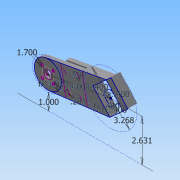
# Autodesk Inventor part: MountSketch
Saved by Autodesk Inventor 2014 SP1 (Build 180222100, 222)
## iProperties
Created: 2014-05-16
Part Number: MountSketch
Material: Generic
Document SubType Name: Modeling
Designer: dliu
Density: 1 g/cm^3
Appearance: Default
Author: dliu
Autodesk Inventor part; units mm, degrees
ref_plane "Back Plane" through (0, 0, -12.7) normal (0, 0, -1) x (-1, 0, 0)
ref_plane "Midplane" through (0, 0, -6.35) normal (0, 0, 1) x (1, 0, 0)
ref_plane "YZ Plane" through (0, 0, 0) normal (1, 0, 0) x (0, 1, 0)
sketch "the Axle" plane through (0, 0, 0) normal (0, 0, 1) x (1, 0, 0)
  line L0 (-30.4731, 63.7704) -> (-43.9693, 51.6183)
  line L1 (-43.9693, 51.6183) -> (-54.1341, 62.9075)
  line L2 (-40.6378, 75.0595) -> (-30.4731, 63.7704)
  line L3 (-30.4731, 63.7704) -> (-12.3121, 63.7704) construction
  arc A0 (-40.6378, 75.0595) -> (-54.1341, 62.9075) centre (-42.9621, 64.0703) ccw
  line L4 (-54.1341, 62.9075) -> (-40.6378, 75.0595) construction
  point P0 (-12.6671, 65.6222)
  dimension "d84" = 18.161
  dimension "d85" = 138
  dimension "d231" = 19.812
  measures "d84" distance of L2.end L1.start
  measures "d85" angle of L0 L3
sketch "Motor Mount Pattern" plane through (0, 0, 0) normal (0, 0, 1) x (1, 0, 0)
  line L0 (-116.3697, 51.2894) -> (-116.3697, 68.9671) construction
  line L1 (-116.3697, 68.9671) -> (-134.0474, 68.9671) construction
  line L2 (-134.0474, 68.9671) -> (-134.0474, 51.2894) construction
  line L3 (-134.0474, 51.2894) -> (-116.3697, 68.9671) construction
  line L4 (-116.3697, 51.2894) -> (-134.0474, 68.9671) construction
  line L5 (-134.0474, 51.2894) -> (-134.0474, 68.9671) construction
  line L6 (-134.0474, 51.2894) -> (-116.3697, 68.9671) construction
  line L7 (-134.0474, 51.2894) -> (-125.2086, 60.1282) construction
  line L8 (-116.3697, 51.2894) -> (-134.0474, 51.2894) construction
  circle A0 centre (-125.2086, 60.1282) radius 6.2
  circle A1 centre (-116.3697, 68.9671) radius 2.25
  circle A2 centre (-134.0474, 68.9671) radius 2.25
  circle A3 centre (-116.3697, 51.2894) radius 2.25
  circle A4 centre (-134.0474, 51.2894) radius 2.25
  circle A5 centre (-116.3697, 68.9671) radius 4.5 construction
  circle A6 centre (-134.0474, 68.9671) radius 4.5 construction
  circle A7 centre (-134.0474, 51.2894) radius 4.5 construction
  circle A8 centre (-116.3697, 51.2894) radius 4.5 construction
  point P0 (-121.7102, 57.8126)
  dimension "d189" = 25
  dimension "d192" = 12.4
  dimension "d193" = 4.5
  dimension "d195" = 9
  measures "d189" distance of L0.start L1.end
  measures "d192" diameter of A0
  measures "d193" diameter of A1
  measures "d195" diameter of A5
sketch "Motor Body Extent" plane through (0, 0, 0) normal (0, 0, 1) x (1, 0, 0)
  circle A0 centre (-176.4641, 62.233) radius 24.5 construction
  dimension "MotorDia" = 49
  measures "MotorDia" diameter of A0
sketch "Block7" plane through (0, 0, 0) normal (0, 0, 1) x (1, 0, 0)
  line L0 (-114.6206, 39.8537) -> (-104.0422, 54.0169) construction
  line L1 (-104.0422, 54.0169) -> (-118.2054, 64.5953) construction
  line L2 (-118.2054, 64.5953) -> (-128.7838, 50.432) construction
  line L3 (-128.7838, 50.432) -> (-104.0422, 54.0169) construction
  line L4 (-114.6206, 39.8537) -> (-118.2054, 64.5953) construction
  line L5 (-128.7838, 50.432) -> (-118.2054, 64.5953) construction
  line L6 (-128.7838, 50.432) -> (-104.0422, 54.0169) construction
  line L7 (-128.7838, 50.432) -> (-116.413, 52.2245) construction
  line L8 (-114.6206, 39.8537) -> (-128.7838, 50.432) construction
  circle A0 centre (-116.413, 52.2245) radius 6.2
  circle A1 centre (-104.0422, 54.0169) radius 2.25
  circle A2 centre (-118.2054, 64.5953) radius 2.25
  circle A3 centre (-114.6206, 39.8537) radius 2.25
  circle A4 centre (-128.7838, 50.432) radius 2.25
  circle A5 centre (-104.0422, 54.0169) radius 4.5 construction
  circle A6 centre (-118.2054, 64.5953) radius 4.5 construction
  circle A7 centre (-128.7838, 50.432) radius 4.5 construction
  circle A8 centre (-114.6206, 39.8537) radius 4.5 construction
  line L9 (-107.5171, 56.2696) -> (-121.6653, 66.8681) construction
  line L10 (-121.6653, 66.8681) -> (-132.2638, 52.7199) construction
  line L11 (-132.2638, 52.7199) -> (-118.1156, 42.1214) construction
  line L12 (-118.1156, 42.1214) -> (-121.6653, 66.8681) construction
  line L13 (-107.5171, 56.2696) -> (-132.2638, 52.7199) construction
  line L14 (-118.1156, 42.1214) -> (-132.2638, 52.7199) construction
  line L15 (-118.1156, 42.1214) -> (-121.6653, 66.8681) construction
  line L16 (-118.1156, 42.1214) -> (-119.8904, 54.4948) construction
  line L17 (-107.5171, 56.2696) -> (-118.1156, 42.1214) construction
  circle A9 centre (-119.8904, 54.4948) radius 6.2
  circle A10 centre (-121.6653, 66.8681) radius 2.25
  circle A11 centre (-132.2638, 52.7199) radius 2.25
  circle A12 centre (-107.5171, 56.2696) radius 2.25
  circle A13 centre (-118.1156, 42.1214) radius 2.25
  circle A14 centre (-121.6653, 66.8681) radius 4.5 construction
  circle A15 centre (-132.2638, 52.7199) radius 4.5 construction
  circle A16 centre (-118.1156, 42.1214) radius 4.5 construction
  circle A17 centre (-107.5171, 56.2696) radius 4.5 construction
  line L18 (-105.811, 55.3186) -> (-120.0113, 65.8472) construction
  line L19 (-120.0113, 65.8472) -> (-130.5399, 51.6469) construction
  line L20 (-130.5399, 51.6469) -> (-116.3396, 41.1183) construction
  line L21 (-116.3396, 41.1183) -> (-120.0113, 65.8472) construction
  line L22 (-105.811, 55.3186) -> (-130.5399, 51.6469) construction
  line L23 (-116.3396, 41.1183) -> (-130.5399, 51.6469) construction
  line L24 (-116.3396, 41.1183) -> (-120.0113, 65.8472) construction
  line L25 (-116.3396, 41.1183) -> (-118.1755, 53.4828) construction
  line L26 (-105.811, 55.3186) -> (-116.3396, 41.1183) construction
  circle A18 centre (-118.1755, 53.4828) radius 6.2
  circle A19 centre (-120.0113, 65.8472) radius 2.25
  circle A20 centre (-130.5399, 51.6469) radius 2.25
  circle A21 centre (-105.811, 55.3186) radius 2.25
  circle A22 centre (-116.3396, 41.1183) radius 2.25
  circle A23 centre (-120.0113, 65.8472) radius 4.5 construction
  circle A24 centre (-130.5399, 51.6469) radius 4.5 construction
  circle A25 centre (-116.3396, 41.1183) radius 4.5 construction
  circle A26 centre (-105.811, 55.3186) radius 4.5 construction
  point P0 (-115.0557, 53.032)
sketch "MotorMountPattern" plane through (0, 0, 0) normal (0, 0, 1) x (1, 0, 0)
  line L0 (-95.4079, 16.8905) -> (-77.7418, 16.8905) construction
  line L1 (-77.7418, 16.8905) -> (-77.7418, 34.5797) construction
  line L2 (-77.7418, 34.5797) -> (-95.4079, 34.5797) construction
  line L3 (-95.4079, 34.5797) -> (-95.4079, 16.8905) construction
  line L4 (-95.4079, 16.8905) -> (-77.7418, 34.5797) construction
  line L5 (-77.7418, 16.8905) -> (-95.4079, 34.5797) construction
  circle A0 centre (-95.4079, 34.5797) radius 2.2
  circle A1 centre (-77.7418, 34.5797) radius 2.2
  circle A2 centre (-77.7418, 16.8905) radius 2.2
  circle A3 centre (-95.4079, 16.8905) radius 2.2
  circle A4 centre (-86.5749, 25.7351) radius 6.35
  point P0 (-86.5749, 25.7351)
  dimension "d197" = 25
  dimension "M4Clearance" = 4.4
  dimension "MotorShaftClearance" = 12.7
  measures "d197" distance of L0.start L1.end
  measures "M4Clearance" diameter of A0
  measures "MotorShaftClearance" diameter of A4
sketch "Base Sketch" plane through (0, 0, 0) normal (0, 0, 1) x (1, 0, 0)
  line L0 (26.8378, -1.0519) -> (-1.7592, -26.8007)
  line L1 (-1.7592, -26.8007) -> (-28.6127, 3.0232)
  line L2 (-28.6127, 3.0232) -> (-0.0158, 28.772)
  line L3 (-0.0158, 28.772) -> (26.8378, -1.0519)
  line L4 (-7.5661, 21.9736) -> (19.2874, -7.8503)
  circle A0 centre (0, 0) radius 41.5 construction
  line L5 (-7.5661, 21.9736) -> (-79.8206, 8.7754)
  line L6 (-97.8004, -38.3626) -> (-71.7823, -35.2304)
  circle A1 centre (-100.3809, -16.9274) radius 21.59
  line L7 (-148.6125, -66.8274) -> (67.2297, -66.8274) construction
  circle A2 centre (-100.3809, -16.9274) radius 24.5 construction
  line L8 (-71.1528, -2.3995) -> (-75.5515, 3.8227)
  line L9 (-65.5155, -27.1154) -> (-69.9143, -20.8933)
  line L10 (-49.848, 2.3791) -> (-54.2467, 8.6013)
  line L11 (-45.6742, -26.5785) -> (-50.073, -20.3564)
  circle A3 centre (-65.5155, -27.1154) radius 2.5527 construction
  line L12 (-45.8783, 14.9754) -> (-37.4622, -31.0988)
  line L13 (-79.8206, 8.7754) -> (-71.7823, -35.2304)
  line L14 (-79.8206, 8.7754) -> (-104.2604, 4.3112)
  line L15 (-71.7823, -35.2304) -> (-1.7592, -26.8007)
  line L16 (12.489, -0.2999) -> (-1.0072, -12.452)
  line L17 (-1.0072, -12.452) -> (-11.172, -1.1629)
  line L18 (2.3243, 10.9892) -> (12.489, -0.2999)
  line L19 (12.489, -0.2999) -> (30.65, -0.2999) construction
  arc A4 (2.3243, 10.9892) -> (-11.172, -1.1629) centre (0, 0) ccw
  line L20 (-11.172, -1.1629) -> (2.3243, 10.9892) construction
  line L21 (-108.9034, -26.0716) -> (-91.2478, -25.4618) construction
  line L22 (-91.2478, -25.4618) -> (-91.8584, -7.7832) construction
  line L23 (-91.8584, -7.7832) -> (-109.514, -8.393) construction
  line L24 (-109.514, -8.393) -> (-108.9034, -26.0716) construction
  line L25 (-108.9034, -26.0716) -> (-91.8584, -7.7832) construction
  line L26 (-91.2478, -25.4618) -> (-109.514, -8.393) construction
  circle A5 centre (-109.514, -8.393) radius 2.2
  circle A6 centre (-91.8584, -7.7832) radius 2.2
  circle A7 centre (-91.2478, -25.4618) radius 2.2
  circle A8 centre (-108.9034, -26.0716) radius 2.2
  circle A9 centre (-100.3809, -16.9274) radius 6.35
  dimension "AxleMargin" = 10.16
  dimension "d97" = 10.16
  dimension "d98" = 10.16
  dimension "d99" = 10.16
  dimension "WheelDia" = 83
  dimension "d157" = 43.18
  dimension "AxleBoardClearance" = 66.8274
  dimension "d233" = 49
  dimension "BoardClearance" = 25.4
  dimension "NomCtrDistance" = 101.7981
  dimension "d258" = 7.62
  dimension "N10Clearance" = 5.1054
  dimension "M4ClearanceDia" = 4.5
  dimension "d211" = 10.8
  dimension "d218" = 9
  constraints: 32 end point, 8 parallel, 7 point on line, 6 perpendicular, 4 centre point, 4 coincident, 4 tangent, 2 point on circle, 1 horizontal, 4 other
  measures "WheelDia" diameter of A0
  measures "d157" diameter of A1
  measures "AxleBoardClearance" distance from line of point (0, 0) L7
  measures "d233" diameter of A2
  measures "BoardClearance" distance edge to line of A2 L7
  measures "NomCtrDistance" distance of point (0, 0) A1.centre
  measures "d258" distance of L10.start L10.end
  measures "N10Clearance" diameter of A3
extrude "Base" add sketch "Base Sketch" against normal blind 15.24 contours L0 L4 L2 L3 | L15 L12 L5 L2 L1 | L15 L13 L5 L12
extrude "Extrusion7" cut sketch "Base Sketch" against normal blind 8.89 contours L15 L13 L5 L12
extrude "Extrusion8" add sketch "Base Sketch" against normal blind 6.35 separate body contours L15 L13 L5 L12 | L6 A1 L14 L13 | A1
sketch "Sketch12" plane through (0, 0, -12.7) normal (0, 0, -1) x (-1, 0, 0)
  line L0 (7.5661, 21.9736) -> (105.9285, 5.8665) projected
  line L1 (100.2333, -36.9167) -> (1.7592, -26.8007) projected
  line L2 (16.1, -21.8905) -> (20.7942, 13.3729)
  line L3 (75.7186, -28.0149) -> (16.1, -21.8905)
  line L4 (20.7942, 13.3729) -> (82.4161, 3.2822)
  line L5 (100.3809, -16.9274) -> (104.4983, -13.952) construction
  line L6 (114.7308, -36.7851) -> (118.8483, -33.8097) construction
  line L7 (90.1484, 5.9057) -> (86.0309, 2.9303) construction
  arc A0 (86.0309, 2.9303) -> (114.7308, -36.7851) centre (100.3809, -16.9274) ccw construction
  arc A1 (118.8483, -33.8097) -> (90.1484, 5.9057) centre (104.4983, -13.952) ccw construction
  line L8 (116.2185, -38.8438) -> (120.336, -35.8684)
  arc A2 (120.336, -35.8684) -> (88.6607, 7.9645) centre (104.4983, -13.952) ccw
  line L9 (88.6607, 7.9645) -> (84.5432, 4.989)
  arc A3 (84.5432, 4.989) -> (82.4161, 3.2822) centre (100.3809, -16.9274) ccw
  arc A4 (75.7186, -28.0149) -> (116.2185, -38.8438) centre (100.3809, -16.9274) ccw
  arc A5 (82.4161, 3.2822) -> (75.7186, -28.0149) centre (100.3809, -16.9274) ccw
  arc A6 (74.798, 4.5297) -> (68.6388, -27.2876) centre (100.3809, -16.9274) ccw
  point P0 (0, 0)
  point P1 (11.172, -1.1629)
  point P2 (102.4396, -15.4397)
  dimension "d178" = 7.62
  dimension "d183" = 6.35
  dimension "d186" = 88.283
  dimension "d187" = 88.283
  dimension "d226" = 6.35
  dimension "d228" = 49
  dimension "d229" = 2.54
  dimension "d251" = 6.35
  dimension "d252" = 2.54
  dimension "d235" = 7.62
  dimension "d236" = 7.62
  constraints: 2 end point, 1 vertical
body "Solid5"
body "Solid4"
body "Solid6"
